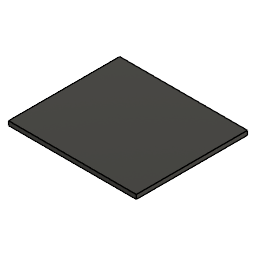
bottom of box (Autodesk Fusion 360 design; units mm, degrees)
part number: 2026-05-12-00-53-29-032
Autodesk Fusion 360 part; units mm, degrees
sketch "Sketch1" plane through (0, 0, 0) normal (0, 0, 1) x (1, 0, 0)
  line L0 (60.1829, 35.0056) -> (-59.0275, 35.0056)
  line L1 (-59.0275, 35.0056) -> (-59.0275, -68.7002)
  line L2 (-59.0275, -68.7002) -> (60.1829, -68.7002)
  line L3 (60.1829, -68.7002) -> (60.1829, 35.0056)
  constraint horizontal L0
  constraint vertical L1
  constraint horizontal L2
  constraint vertical L3
extrude "Extrude1" add sketch "Sketch1" against normal blind 3.994
move_body "Move1" bodies 1 to x (1, 0, 0) y (0, 1, 0) z (0, 0, 1) at (0, 0, 13)
